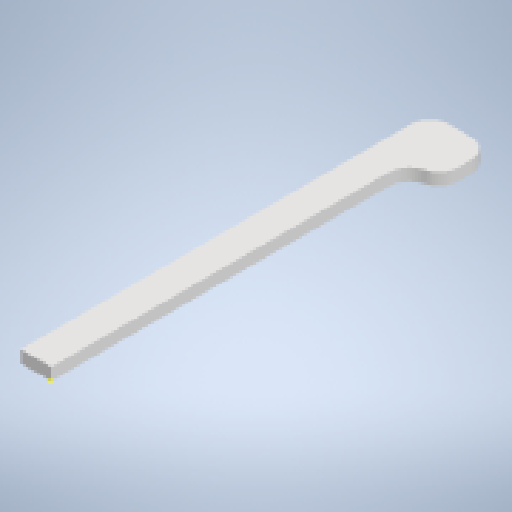
# Autodesk Inventor part: MoveableBarRound
Saved by Autodesk Inventor 2024 (Build 280153000, 153)
## iProperties
Created: 2024-10-03
Part Number: MoveableBarRound
Material: Generic
Document SubType Name: Modeling
Designer: xxred
Density: 1 g/cm^3
Appearance: Default
Author: xxred
Autodesk Inventor part; units mm, degrees
ref_plane "YZ Plane" through (0, 0, 0) normal (1, 0, 0) x (0, 1, 0)
ref_plane "XZ Plane" through (0, 0, 0) normal (0, 1, 0) x (-1, 0, 0)
ref_plane "XY Plane" through (0, 0, 0) normal (0, 0, 1) x (1, 0, 0)
sketch "Sketch1" plane through (0, 0, 0) normal (0, 1, 0) x (-1, 0, 0)
  point P0 (0, 0)
sketch "Sketch2" plane through (0, 0, 0) normal (0, 1, 0) x (-1, 0, 0)
  line L0 (0, 0) -> (3, 0)
  line L1 (3, 0) -> (3, -40)
  line L2 (3, -40) -> (0, -40)
  line L3 (0, -40) -> (0, 0)
  line L4 (0, -40) -> (-3, -40)
  line L5 (-3, -40) -> (-3, -35)
  line L6 (-3, -35) -> (0, -35)
  line L7 (0, -35) -> (0, -40)
  point P0 (0, -35)
  dimension "d0" = 3
  dimension "d1" = 40
  dimension "d4" = 3
  dimension "d5" = 5
  constraints: 16 end point, 4 parallel, 2 horizontal, 2 perpendicular
  measures "d0" distance of L1.end L2.end
  measures "d1" distance of L0.end L1.end
  measures "d4" distance of L5.end L6.end
  measures "d5" distance of L4.end L5.end
extrude "Extrusion1" add sketch "Sketch2" along normal blind 1.2
fillet "Fillet1" radius 2 4 edges at (0, 0.6, -35) (3, 0.6, -35) (3, 0.6, -40) (-3, 0.6, -40)
body "Solid1"
